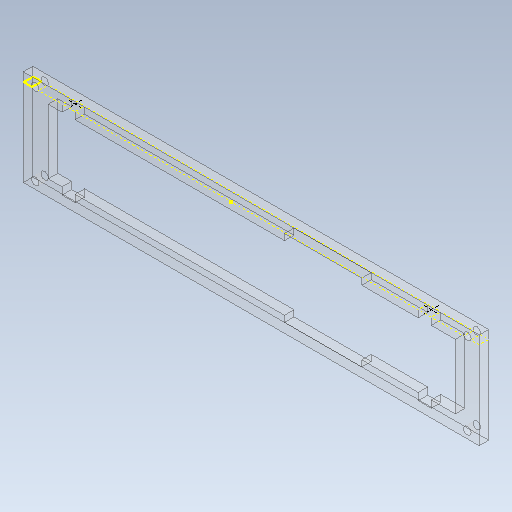
# Autodesk Inventor part: Template-Fixture-Mid
Saved by Autodesk Inventor 2021 (Build 250183000, 183)
## iProperties
Created: 2020-06-16
Part Number: Template-Fixture-Mid
Material: Polycarbonate, Clear
Document SubType Name: Modeling
Designer: lucas
Density: 1.2 g/cm^3
Appearance: Polycarbonate - Clear
Project: 4Wire-FDM
Author: lucas
Revision Number: RLS_004
Autodesk Inventor part; units mm, degrees
ref_plane "YZ Plane" through (0, 0, 0) normal (1, 0, 0) x (0, 1, 0)
ref_plane "XZ Plane" through (0, 0, 0) normal (0, 1, 0) x (-1, 0, 0)
ref_plane "XY Plane" through (0, 0, 0) normal (0, 0, 1) x (1, 0, 0)
sketch "Sketch1" plane through (0, 0, 0) normal (0, 0, 1) x (1, 0, 0)
  line L0 (93.3916, -12.6) -> (93.3916, 12.6)
  line L1 (53.9763, -12.6) -> (93.3916, -12.6)
  line L2 (53.9763, -15.2) -> (53.9763, -12.6)
  line L3 (38.2753, -15.2) -> (53.9763, -15.2)
  line L4 (38.2753, -15.2) -> (23.4296, -15.2)
  line L5 (23.4296, -12.6) -> (23.4296, -15.2)
  line L6 (-76.0546, -12.6) -> (23.4296, -12.6)
  line L7 (23.4296, 12.6) -> (-76.0546, 12.6)
  line L8 (23.4296, 15.2) -> (23.4296, 12.6)
  line L9 (-76.0546, 12.6) -> (-76.0546, -12.6)
  line L10 (-70.1, 10) -> (-66.9, 10)
  line L11 (-66.9, -10) -> (-70.1, -10)
  line L12 (23.4296, 15.2) -> (53.9763, 15.2)
  line L13 (53.9763, 15.2) -> (53.9763, 12.6)
  line L14 (53.9763, 12.6) -> (93.3916, 12.6)
  line L15 (-77.0546, 13.6) -> (22.4296, 13.6)
  line L16 (22.4296, 13.6) -> (22.4296, 16.2)
  line L17 (22.4296, 16.2) -> (54.9763, 16.2)
  line L18 (54.9763, 16.2) -> (54.9763, 13.6)
  line L19 (54.9763, 13.6) -> (94.3916, 13.6)
  line L20 (94.3916, 13.6) -> (94.3916, -13.6)
  line L21 (94.3916, -13.6) -> (54.9763, -13.6)
  line L22 (54.9763, -13.6) -> (54.9763, -16.2)
  line L23 (54.9763, -16.2) -> (38.2753, -16.2)
  line L24 (38.2753, -16.2) -> (22.4296, -16.2)
  line L25 (22.4296, -16.2) -> (22.4296, -13.6)
  line L26 (22.4296, -13.6) -> (-77.0546, -13.6)
  line L27 (-77.0546, -13.6) -> (-77.0546, 13.6)
  line L28 (22.4296, -16.2) -> (22.4296, -20.2) construction
  line L29 (22.4296, -20.2) -> (-87.5704, -20.2)
  line L30 (-87.5704, -20.2) -> (-87.5704, 20.2)
  line L31 (-87.5704, 20.2) -> (22.4296, 20.2)
  line L32 (104.4296, -20.2) -> (22.4296, -20.2)
  line L33 (22.4296, 20.2) -> (104.4296, 20.2)
  line L34 (104.4296, 20.2) -> (104.4296, -20.2)
  circle A0 centre (-82.5704, 17.2) radius 1.6
  circle A1 centre (-82.5704, -17.2) radius 1.6
  circle A2 centre (99.4296, 17.2) radius 1.6
  circle A3 centre (99.4296, -17.2) radius 1.6
  dimension "d0" = 1
  dimension "d1" = 4
  dimension "d2" = 110
  dimension "d3" = 40.4
  dimension "d5" = 82
  dimension "d18" = 5
  dimension "d19" = 5
  dimension "d20" = 3
  dimension "d21" = 3
  dimension "d22" = 5
  dimension "d23" = 3
  dimension "d24" = 5
  dimension "d25" = 3
  constraints: 70 end point, 7 perpendicular, 4 centre point, 2 horizontal, 1 parallel, 1 point on line, 1 vertical, 12 other
  measures "d0" distance between parallel lines of L7 L15
  measures "d1" distance of L24.end L28.end
  measures "d2" distance of L28.end L29.end
  measures "d3" distance of L29.end L30.end
  measures "d5" distance of L31.end L33.end
  measures "d18" distance from line of L30 A0.centre
  measures "d19" distance from line of L30 A1.centre
  measures "d20" distance from line of L29 A1.centre
  measures "d21" distance from line of L31 A0.centre
  measures "d22" distance from line of L34 A3.centre
  measures "d23" distance from line of L32 A3.centre
  measures "d24" distance from line of L34 A2.centre
  measures "d25" distance from line of L33 A2.centre
extrude "Extrusion1" add sketch "Sketch1" against normal blind 4 contours L29 L30 L31 L33 L34 L32
sketch "Sketch2" plane through (0, 0, 0) normal (0, 0, 1) x (1, 0, 0)
  line L0 (79.9, -10) -> (83.1, -10) construction
  line L1 (83.1, 10) -> (79.9, 10) construction
  line L2 (-66.9, -10) -> (-70.1, -10) construction
  line L3 (-70.1, 10) -> (-66.9, 10) construction
  line L4 (81.5, -10) -> (81.5, -13.6) construction
  line L5 (94.3916, -13.6) -> (54.9763, -13.6) projected
  line L6 (81.5, 10) -> (81.5, 13.6) construction
  line L7 (54.9763, 13.6) -> (94.3916, 13.6) projected
  line L8 (-68.5, -10) -> (-68.5, -13.6) construction
  line L9 (22.4296, -13.6) -> (-77.0546, -13.6) projected
  line L10 (-68.5, 10) -> (-68.5, 13.6) construction
  line L11 (-77.0546, 13.6) -> (22.4296, 13.6) projected
  line L12 (84.25, -10.6) -> (78.75, -10.6)
  line L13 (78.75, -10.6) -> (78.75, -16.6)
  line L14 (78.75, -16.6) -> (84.25, -16.6)
  line L15 (84.25, -16.6) -> (84.25, -10.6)
  line L16 (84.25, -10.6) -> (78.75, -16.6) construction
  line L17 (78.75, -10.6) -> (84.25, -16.6) construction
  line L18 (84.25, 10.6) -> (78.75, 10.6)
  line L19 (78.75, 10.6) -> (78.75, 16.6)
  line L20 (78.75, 16.6) -> (84.25, 16.6)
  line L21 (84.25, 16.6) -> (84.25, 10.6)
  line L22 (84.25, 10.6) -> (78.75, 16.6) construction
  line L23 (78.75, 10.6) -> (84.25, 16.6) construction
  line L24 (-65.75, 10.6) -> (-71.25, 10.6)
  line L25 (-71.25, 10.6) -> (-71.25, 16.6)
  line L26 (-71.25, 16.6) -> (-65.75, 16.6)
  line L27 (-65.75, 16.6) -> (-65.75, 10.6)
  line L28 (-65.75, 10.6) -> (-71.25, 16.6) construction
  line L29 (-71.25, 10.6) -> (-65.75, 16.6) construction
  line L30 (-65.75, -10.6) -> (-71.25, -10.6)
  line L31 (-71.25, -10.6) -> (-71.25, -16.6)
  line L32 (-71.25, -16.6) -> (-65.75, -16.6)
  line L33 (-65.75, -16.6) -> (-65.75, -10.6)
  line L34 (-65.75, -10.6) -> (-71.25, -16.6) construction
  line L35 (-71.25, -10.6) -> (-65.75, -16.6) construction
  point P0 (0, 0)
  point P1 (-71.25, 13.6)
  point P2 (-65.75, 13.6)
  point P3 (-65.75, -13.6)
  point P4 (-71.25, -13.6)
  point P5 (78.75, 13.6)
  point P6 (84.25, 13.6)
  point P7 (84.25, -13.6)
  point P8 (78.75, -13.6)
  dimension "d8" = 5.5
  dimension "d9" = 6
  dimension "d10" = 5.5
  dimension "d11" = 6
  dimension "d12" = 5.5
  dimension "d13" = 6
  dimension "d14" = 5.5
  dimension "d15" = 6
  constraints: 64 end point, 12 midpoint, 9 parallel, 6 point on line, 4 perpendicular, 1 vertical
  measures "d8" distance of L12.start L12.end
  measures "d9" distance of L13.end L12.end
  measures "d10" distance of L18.start L18.end
  measures "d11" distance of L18.end L19.end
  measures "d12" distance of L24.start L24.end
  measures "d13" distance of L24.end L25.end
  measures "d14" distance of L30.start L30.end
  measures "d15" distance of L31.end L30.end
extrude "Extrusion2" cut sketch "Sketch2" against normal blind 4 contours L15 L14 L13 L5 | L19 L20 L21 L7 | L33 L32 L31 L9 | L25 L26 L27 L11
sketch "Sketch4" plane through (-71.25, 16.6, 0) normal (0, -1, 0) x (1, 0, 0)
  line L0 (0, 0) -> (0, -4) construction
  line L1 (5.5, -4) -> (0, -4) construction
  line L2 (150, -4) -> (5.5, -4) construction
  line L3 (155.5, -4) -> (150, -4) construction
  line L4 (169.1963, -4) -> (155.5, -4) construction
  line L5 (169.1963, 0) -> (169.1963, -4) construction
  line L6 (155.5, 0) -> (169.1963, 0) construction
  line L7 (155.5, -4) -> (155.5, 0) construction
  line L8 (0, 0) -> (5.5, 0) construction
  line L9 (-9.8372, 0) -> (0, 0) construction
  line L10 (-9.8372, -4) -> (-9.8372, 0) construction
  line L11 (0, -4) -> (-9.8372, -4) construction
  line L12 (5.5, -4) -> (5.5, 0) construction
  line L13 (150, 0) -> (150, -4) construction
  line L14 (5.5, 0) -> (150, 0) construction
  line L15 (150, 0) -> (155.5, 0) construction
  line L16 (175.6796, -4) -> (172.1628, -4) construction
  line L17 (172.1628, -4) -> (172.1628, 0) construction
  line L18 (172.1628, 0) -> (175.6796, 0) construction
  line L19 (175.6796, 0) -> (175.6796, -4) construction
  line L20 (-12.8037, -4) -> (-16.3204, -4) projected
  line L21 (-16.3204, -4) -> (-16.3204, 0) projected
  line L22 (-16.3204, 0) -> (-12.8037, 0) projected
  line L23 (-12.8037, 0) -> (-12.8037, -4) projected
  line L24 (0, 0) -> (5.5, 0) construction
  line L25 (2.75, 0) -> (2.75, -2.75) construction
  line L26 (150, 0) -> (155.5, 0) construction
  line L27 (152.75, 0) -> (152.75, -2.75) construction
  point P0 (71.25, 0)
  dimension "d26" = 2.75
  dimension "d27" = 2.75
  constraints: 4 end point, 2 coincident, 2 midpoint, 2 vertical
  measures "d26" distance of L25.start L25.end
  measures "d27" distance of L27.start L27.end
body "Solid1"
